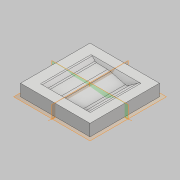
# Autodesk Inventor part: Placa - Abrasión
Saved by Autodesk Inventor 2017 (Build 210142000, 142)
## iProperties
Part Number: Placa - Abrasión
Material: Genérico
Document SubType Name: Modeling
Designer: franc
Density: 1 g/cm^3
Appearance: Valor por defecto
Author: franc
Autodesk Inventor part; units mm, degrees
sketch "Boceto1" plane through (0, 0, 0) normal (0, 0, 1) x (1, 0, 0)
  line L0 (-75, 75) -> (75, 75)
  line L1 (75, 75) -> (75, -75)
  line L2 (75, -75) -> (-75, -75)
  line L3 (-75, -75) -> (-75, 75)
  line L4 (-75, 75) -> (75, -75) construction
  line L5 (75, 75) -> (-75, -75) construction
  point P0 (0, 0)
  dimension "d0" = 150
  dimension "d1" = 150
  constraints: 12 end point, 2 midpoint, 2 parallel, 1 horizontal, 1 perpendicular
  measures "d0" distance of L1.end L2.end
  measures "d1" distance of L0.end L1.end
extrude "Extrusión1" add sketch "Boceto1" along normal blind 25.4
sketch "Boceto2" plane through (0, 0, 0) normal (0, 1, 0) x (-1, 0, 0)
  line L0 (50.8205, 25.4) -> (-38.2556, 25.4)
  line L1 (-75, 0) -> (-75, 25.4) projected
  line L2 (-35.1795, 15.4) -> (8.2824, 20.4)
  line L3 (8.2824, 20.4) -> (37.9796, 20.9)
  line L4 (50.8205, 25.4) -> (37.9796, 20.9)
  line L5 (-75, 25.4) -> (75, 25.4) projected
  line L6 (-35.1795, 15.4) -> (-52.5, 25.4)
  line L7 (-38.2556, 25.4) -> (-52.5, 25.4)
  point P0 (0, 0)
  dimension "d18" = 5
  dimension "d19" = 4.5
  dimension "d20" = 10
  dimension "d21" = 20
  dimension "d22" = 86
  dimension "d23" = 22.5
  constraints: 12 end point, 1 point on line
  measures "d18" distance from line of L2.end L0
  measures "d19" distance from line of L0 L3.end
  measures "d20" distance from line of L5 L2.start
  measures "d21" distance of L2.start L6.end
  measures "d22" horizontal distance of L0.start L2.start
  measures "d23" distance from line of L1 L6.end
extrude "Extrusión3" cut sketch "Boceto2" against normal blind 45
fillet "Empalme8" radius 12 2 edges at (35.1795, -22.5, 15.4) (-37.9796, -22.5, 20.9)
chamfer "Chaflán1" distance 9.625 angle 45 1 edges at (0.8397, -45, 25.4)
mirror "Simetría1" about plane through (0, 0, 0) normal (0, 1, 0) of "Extrusión3", "Empalme8", "Chaflán1"
fillet "Empalme9" radius 10 2 edges at (-50.8205, 0, 25.4) (52.5, 0, 25.4)
fillet "Empalme10" radius 75.25 1 edges at (-8.2824, 0, 20.4)
